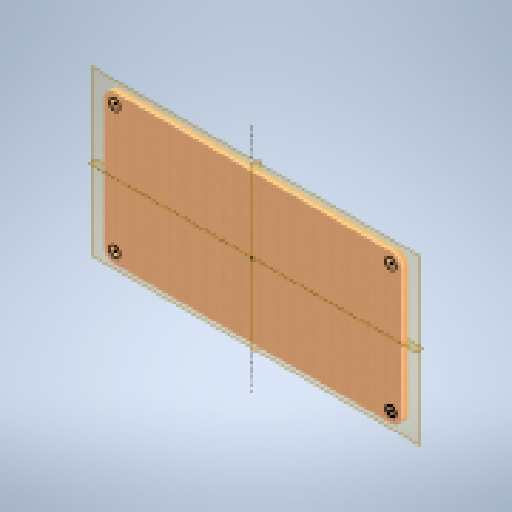
# Autodesk Inventor part: Sessao_02_04_002_001
Saved by Autodesk Inventor 2026 (Build 300175000, 175)
## iProperties
Created: 2025-04-02
Part Number: Sessao_02_04_002_001
Material: Wood (Cherry)
Document SubType Name: Modeling
Designer: Carlos Dias
Density: 0.63 g/cm^3
Appearance: Cherry - Natural Low Gloss
Mass: 18417.2 g
Surface Area: 20904.6 cm^2
Volume: 29233.7 cm^3
Author: Carlos Dias
Autodesk Inventor part; units mm, degrees
sketch "Sketch1" plane through (0, 0, 0) normal (0, 0, 1) x (1, 0, 0)
  line L0 (-700, 350) -> (700, 350)
  line L1 (700, 350) -> (700, -350)
  line L2 (700, -350) -> (-700, -350)
  line L3 (-700, -350) -> (-700, 350)
  line L4 (-700, 350) -> (700, -350) construction
  line L5 (700, 350) -> (-700, -350) construction
  point P0 (0, 0)
  point P1 (0, 0)
  dimension "d1" = 1400
  dimension "d2" = 700
  constraints: 12 end point, 2 midpoint, 2 parallel, 1 coincident, 1 horizontal, 1 perpendicular
  measures "d1" distance of L0.start L0.end
  measures "d2" distance of L0.end L1.end
extrude "Extrusion1" add sketch "Sketch1" along normal mid plane 30
fillet "Fillet1" radius 50 4 edges at (700, 350, 0) (-700, 350, 0) (700, -350, 0) (-700, -350, 0)
sketch "Sketch2" plane through (0, 0, 15) normal (0, 0, 1) x (1, 0, 0)
  circle A0 centre (650, -300) radius 25.4
  line L0 (-737.5381, 0) -> (737.5381, 0) construction
  circle A1 centre (650, 300) radius 25.4
  line L1 (0, -555.4788) -> (0, 555.4788) construction
  circle A2 centre (-650, -300) radius 25.4
  circle A3 centre (-650, 300) radius 25.4
  circle A4 centre (650, -300) radius 19.6
  circle A5 centre (-650, -300) radius 19.6
  circle A6 centre (650, 300) radius 19.6
  circle A7 centre (-650, 300) radius 19.6
  point P0 (0, 0)
  point P1 (0, 0)
  point P2 (0, 0)
  dimension "d6" = 50.8
  dimension "d7" = 650
  dimension "d8" = 300
  dimension "d15" = 5.8
  constraints: 8 centre point, 6 equal radius, 5 coincident, 4 end point, 2 midpoint, 1 horizontal, 1 vertical, 6 other
  measures "d6" diameter of A0
  measures "d7" horizontal distance of point (0, 0) A0.centre
  measures "d8" vertical distance of point (0, 0) A0.centre
  measures "d15" radial gap between concentric circles of A0 A4
extrude "Extrusion2" cut sketch "Sketch2" against normal blind 15
body "Solid1"
